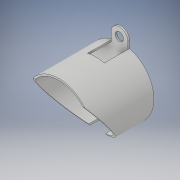
# Autodesk Inventor part: CatWaterSensorCase
Saved by Autodesk Inventor 2018 (Build 220112000, 112)
## iProperties
Created: 2020-11-19
Part Number: CatWaterSensorCase
Material: Generic
Document SubType Name: Modeling
Designer: dangl
Density: 1 g/cm^3
Appearance: Default
Author: dangl
Autodesk Inventor part; units mm, degrees
ref_plane "YZ Plane" through (0, 0, 0) normal (1, 0, 0) x (0, 1, 0)
ref_plane "XZ Plane" through (0, 0, 0) normal (0, 1, 0) x (-1, 0, 0)
ref_plane "XY Plane" through (0, 0, 0) normal (0, 0, 1) x (1, 0, 0)
sketch "Sketch1" plane through (0, 0, 0) normal (0, 0, 1) x (1, 0, 0)
  circle A0 centre (0, 0) radius 18.5
  circle A1 centre (0, 0) radius 19.5
  line L0 (0, 0) -> (0, 25.1943)
  arc A2 (5, 23) -> (-5, 23) centre (0, 23) ccw
  line L1 (5, 23) -> (5, 18.8481)
  line L2 (-5, 23) -> (-5, 18.8481)
  circle A3 centre (0, 23) radius 2.5
  point P0 (-5, 25.1943)
  point P1 (5, 25.1943)
  dimension "d0" = 37
  dimension "d1" = 1
  dimension "d16" = 10
  dimension "d17" = 23
  dimension "d18" = 5
  constraints: 6 end point, 4 centre point, 4 point on circle, 3 coincident, 2 vertical, 1 point on line, 1 symmetric about line
  measures "d0" diameter of A0
  measures "d1" radial gap between concentric circles of A0 A1
  measures "d16" diameter of A2
  measures "d17" distance of point (0, 0) A2.centre
  measures "d18" diameter of A3
extrude "Extrusion1" add sketch "Sketch1" against normal blind 1 contours A0 | A1
extrude "Extrusion2" add sketch "Sketch1" along normal blind 36 contours A1
sketch "Sketch2" plane through (0, 0, 0) normal (1, 0, 0) x (0, 1, 0)
  line L0 (19.5, 36) -> (-19.5, 36) projected
  line L1 (12, 36) -> (-19.5, 12)
  line L2 (-19.5, 36) -> (-19.5, -1) projected
  line L3 (12, 36) -> (19.5, 36)
  line L4 (-19.5, 12) -> (-19.5, -1)
  line L5 (-19.5, -1) -> (19.5, -1) projected
  line L6 (-19.5, -1) -> (19.5, -1)
  line L7 (19.5, -1) -> (19.5, 36)
  point P0 (0, 0)
  dimension "d7" = 12
  dimension "d8" = 12
  constraints: 10 end point, 2 collinear, 2 point on line, 1 horizontal, 1 perpendicular
  measures "d7" horizontal distance of point (0, 0) L1.start
  measures "d8" vertical distance of point (0, 0) L1.end
extrude "Extrusion3" cut sketch "Sketch2" along normal mid plane 50 contours L1 L2 L0
sketch "Sketch3" plane through (0, 0, 0) normal (0, 1, 0) x (-1, 0, 0)
  line L0 (18.5, 0) -> (-18.5, 0) projected
  line L1 (5, 0) -> (-5, 0)
  line L2 (-5, 0) -> (-5, 14)
  line L3 (-5, 14) -> (5, 14)
  line L4 (5, 14) -> (5, 0)
  point P0 (0, 0)
  dimension "d11" = 5
  dimension "d12" = 10
  dimension "d13" = 14
  constraints: 8 end point, 2 parallel, 1 horizontal, 1 perpendicular, 1 point on line
  measures "d11" distance from line of point (0, 0) L4
  measures "d12" distance of L2.end L3.end
  measures "d13" distance of L1.end L2.end
extrude "Extrusion4" cut sketch "Sketch3" along normal mid plane 50
extrude "Extrusion5" add sketch "Sketch1" against normal blind 1 contours A1 L2 A2 L1
body "Solid1"
